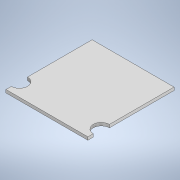
# Autodesk Inventor part: Cover
Saved by Autodesk Inventor 2022.3 (Build 263350000, 350)
## iProperties
Created: 2023-04-12
Part Number: Cover
Material: Generic
Document SubType Name: Modeling
Designer: Siggi
Density: 1 g/cm^3
Appearance: Default
Author: Siggi
Autodesk Inventor part; units mm, degrees
ref_plane "YZ Plane" through (0, 0, 0) normal (1, 0, 0) x (0, 1, 0)
ref_plane "XZ Plane" through (0, 0, 0) normal (0, 1, 0) x (-1, 0, 0)
ref_plane "XY Plane" through (0, 0, 0) normal (0, 0, 1) x (1, 0, 0)
sketch "Sketch2" plane through (0, 0, 0) normal (0, 1, 0) x (-1, 0, 0)
  line L0 (0, 0) -> (-137, 0)
  line L1 (-137, 144) -> (0, 144)
  line L2 (0, 144) -> (-137, 144)
  line L3 (-137, 144) -> (-137, 134.2279)
  line L4 (0, 135) -> (0, 144)
  arc A0 (0, 135) -> (0, 108) centre (0, 121.5) ccw
  line L5 (-137, 0) -> (-137, 108.7721)
  line L6 (-137, 134.2279) -> (-137, 144)
  line L7 (0, 144) -> (0, 135)
  line L8 (0, 108) -> (0, 0)
  arc A1 (-137, 108) -> (-137, 135) centre (-137, 121.5) ccw
  point P0 (-13.5, 121.5)
  point P1 (-123.5, 121.5)
  dimension "d0" = 137
  dimension "d4" = 27
  dimension "d6" = 27
  dimension "d7" = 110
  dimension "d8" = 22.5
  constraints: 18 end point, 6 parallel, 6 point on circle, 3 perpendicular, 2 centre point, 2 horizontal, 2 point on line
  measures "d0" distance of L1.start L1.end
  measures "d4" diameter of A0
  measures "d6" diameter of A1
  measures "d7" distance of point (-13.5, 121.5) point (-123.5, 121.5)
  measures "d8" distance of L1.start A1.centre
extrude "Extrusion1" add sketch "Sketch2" along normal blind 5
body "Solid1"
